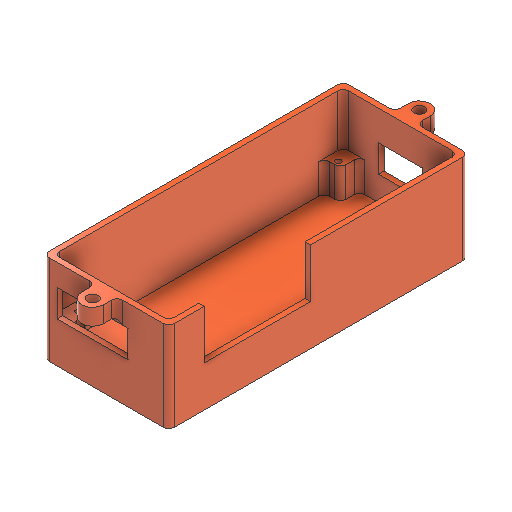
# Autodesk Inventor part: StereoPiBracket
Saved by Autodesk Inventor 2025.2 (Build 292293000, 293)
## iProperties
Created: 2024-08-19
Part Number: StereoPiBracket
Material: Generic
Document SubType Name: Modeling
Designer: 16366081
Density: 1 g/cm^3
Appearance: Default
Author: 16366081
Autodesk Inventor part; units mm, degrees
ref_plane "YZ Plane" through (0, 0, 0) normal (1, 0, 0) x (0, 1, 0)
ref_plane "XZ Plane" through (0, 0, 0) normal (0, 1, 0) x (-1, 0, 0)
ref_plane "XY Plane" through (0, 0, 0) normal (0, 0, 1) x (1, 0, 0)
sketch "Sketch1" plane through (0, 0, 0) normal (0, 1, 0) x (-1, 0, 0)
  line L0 (-23, 55) -> (23, 55)
  line L1 (23, 55) -> (23, -55)
  line L2 (23, -55) -> (-23, -55)
  line L3 (-23, -55) -> (-23, 55)
  line L4 (-23, 55) -> (23, -55) construction
  line L5 (23, 55) -> (-23, -55) construction
  point P0 (0, 0)
  dimension "d0" = 46
  dimension "d1" = 110
  constraints: 12 end point, 2 midpoint, 2 parallel, 1 horizontal, 1 perpendicular
  measures "d0" distance of L1.end L2.end
  measures "d1" distance of L0.end L1.end
extrude "Extrusion1" add sketch "Sketch1" along normal blind 3
sketch "Sketch2" plane through (0, 3, 0) normal (0, 1, 0) x (1, 0, 0)
  line L0 (-23, 55) -> (-23, -55) projected
  line L1 (23, -55) -> (-23, -55)
  line L2 (-23, -55) -> (-23, 55)
  line L3 (-23, 55) -> (23, 55)
  line L4 (23, 55) -> (23, -55)
  line L5 (23, -55) -> (-23, 55) construction
  line L6 (-23, -55) -> (23, 55) construction
  line L7 (21, -53) -> (-21, -53)
  line L8 (-21, -53) -> (-21, 53)
  line L9 (-21, 53) -> (21, 53)
  line L10 (21, 53) -> (21, -53)
  line L11 (21, -53) -> (-21, 53) construction
  line L12 (-21, -53) -> (21, 53) construction
  point P0 (0, 0)
  dimension "d4" = 42
  dimension "d5" = 106
  constraints: 24 end point, 4 midpoint, 4 parallel, 2 horizontal, 2 perpendicular
  measures "d4" distance of L8.end L9.end
  measures "d5" distance of L7.end L8.end
extrude "Extrusion2" add sketch "Sketch2" along normal blind 30
sketch "Sketch5" plane through (0, 33, 0) normal (0, 1, 0) x (1, 0, 0)
  line L0 (23, 55) -> (-23, 55) projected
  line L1 (23, -55) -> (23, 55) projected
  line L2 (-23, 55) -> (-23, -55) projected
  line L3 (21, 53) -> (21, -53) projected
  line L4 (21, -42) -> (23, -42)
  line L5 (23, -42) -> (23, -3)
  line L6 (23, -3) -> (21, -3)
  line L7 (21, -3) -> (21, -42)
  line L8 (-23, -55) -> (23, -55) projected
  point P0 (0, 0)
  point P1 (22, -42)
  point P2 (22, -3)
  dimension "d24" = 13
  dimension "d25" = 58
  constraints: 8 end point, 2 midpoint, 2 parallel, 2 point on line, 1 horizontal, 1 perpendicular
  measures "d24" distance from line of L8 point (22, -42)
  measures "d25" distance from line of L0 point (22, -3)
extrude "Extrusion5" cut sketch "Sketch5" against normal blind 18 contours L1 L4 L3 L6
sketch "Sketch6" plane through (23, 0, -55) normal (0, 0, -1) x (-1, 0, 0)
  line L0 (15, 22) -> (31, 22)
  line L1 (31, 22) -> (31, 12)
  line L2 (31, 12) -> (15, 12)
  line L3 (15, 12) -> (15, 22)
  line L4 (46, 0) -> (46, 33) projected
  line L5 (0, 0) -> (46, 0) projected
  point P0 (23, 0)
  dimension "d28" = 16
  dimension "d29" = 15
  dimension "d30" = 10
  dimension "d32" = 12
  constraints: 8 end point, 2 parallel, 1 horizontal, 1 perpendicular
  measures "d28" distance of L0.start L0.end
  measures "d29" distance from line of L4 L1.end
  measures "d30" distance of L2.end L0.start
  measures "d32" distance between parallel lines of L5 L2
extrude "Extrusion6" cut sketch "Sketch6" against normal blind 15
sketch "Sketch7" plane through (-23, 0, 55) normal (0, 0, 1) x (1, 0, 0)
  line L0 (5, 25) -> (31, 25)
  line L1 (31, 25) -> (31, 15)
  line L2 (31, 15) -> (5, 15)
  line L3 (5, 15) -> (5, 25)
  line L4 (0, 0) -> (0, 33) projected
  line L5 (0, 0) -> (46, 0) projected
  point P0 (23, 0)
  dimension "d35" = 5
  dimension "d36" = 10
  dimension "d37" = 15
  dimension "d38" = 26
  constraints: 8 end point, 2 parallel, 1 horizontal, 1 perpendicular
  measures "d35" distance between parallel lines of L4 L3
  measures "d36" distance of L2.end L0.start
  measures "d37" distance between parallel lines of L5 L2
  measures "d38" distance of L1.end L2.end
extrude "Extrusion7" cut sketch "Sketch7" against normal blind 15
sketch "Sketch9" plane through (0, 33, 0) normal (0, 1, 0) x (1, 0, 0)
  circle A0 centre (0, -60) radius 2
  line L0 (-23, -55) -> (23, -55) projected
  line L1 (4, -55) -> (-4, -55)
  line L2 (-4, -55) -> (-4, -60)
  line L3 (4, -60) -> (4, -55)
  arc A1 (-4, -60) -> (4, -60) centre (0, -60) ccw
  circle A2 centre (0, 60) radius 2
  line L4 (23, 55) -> (-23, 55) projected
  line L5 (4, 55) -> (-4, 55)
  line L6 (-4, 55) -> (-4, 60)
  line L7 (4, 60) -> (4, 55)
  arc A3 (4, 60) -> (-4, 60) centre (0, 60) ccw
  point P0 (0, 0)
  point P1 (0, -55)
  point P2 (0, -55)
  point P3 (0, 55)
  point P4 (0, 55)
  point P5 (0, 55)
  dimension "d77" = 4
  dimension "d78" = 5
  dimension "d79" = 8
  dimension "d80" = 4
  dimension "d81" = 4
  dimension "d82" = 4
  dimension "d83" = 5
  dimension "d84" = 8
  dimension "d85" = 4
  constraints: 12 end point, 5 midpoint, 4 centre point, 4 point on circle, 2 coincident, 2 horizontal, 2 parallel, 2 perpendicular, 2 point on line, 1 tangent, 1 vertical alignment
  measures "d77" diameter of A0
  measures "d78" distance of point (0, -55) A0.centre
  measures "d79" distance of L1.start L1.end
  measures "d80" distance of point (0, -55) L1.start
  measures "d81" radius of A1
  measures "d82" diameter of A2
  measures "d83" distance of point (0, 55) A2.centre
  measures "d84" distance of L5.end L5.start
  measures "d85" distance of L5.start point (0, 55)
extrude "Extrusion10" add sketch "Sketch9" against normal blind 6
fillet "Fillet2" radius 2 6 edges at (-4, 30, -55) (4, 30, -55) (-4, 30, 55) (4, 30, 55) (0, 27, -55) (0, 27, 55)
sketch "Sketch11" plane through (0, 3, 0) normal (0, 1, 0) x (1, 0, 0)
  circle A0 centre (-17.5, 47.75) radius 1
  circle A1 centre (17.5, 47.75) radius 1
  circle A2 centre (-17.5, -47.75) radius 1
  circle A3 centre (17.5, -47.75) radius 1
  line L0 (-21, 53) -> (-21, -53) projected
  line L1 (-21, 53) -> (-15, 53)
  line L2 (-15, 53) -> (-15, 46)
  line L3 (-15, 46) -> (-21, 46)
  line L4 (-21, 46) -> (-21, 53)
  line L5 (21, 53) -> (-21, 53) projected
  line L6 (21, 53) -> (15, 53)
  line L7 (15, 53) -> (15, 46)
  line L8 (15, 46) -> (21, 46)
  line L9 (21, 46) -> (21, 53)
  line L10 (-21, -53) -> (-15, -53)
  line L11 (-15, -53) -> (-15, -46)
  line L12 (-15, -46) -> (-21, -46)
  line L13 (-21, -46) -> (-21, -53)
  line L14 (21, -53) -> (15, -53)
  line L15 (15, -53) -> (15, -46)
  line L16 (15, -46) -> (21, -46)
  line L17 (21, -46) -> (21, -53)
  point P0 (0, 0)
  dimension "d95" = 2
  dimension "d96" = 2
  dimension "d97" = 2
  dimension "d98" = 2
  dimension "d99" = 95.5
  dimension "d100" = 35
  dimension "d101" = 47.75
  dimension "d102" = 17.5
  dimension "d103" = 6
  dimension "d104" = 7
  dimension "d105" = 6
  dimension "d106" = 7
  dimension "d107" = 6
  dimension "d108" = 7
  dimension "d109" = 6
  dimension "d110" = 7
  constraints: 32 end point, 8 parallel, 4 centre point, 4 horizontal, 4 perpendicular, 2 horizontal alignment, 2 point on line, 2 vertical alignment
  measures "d95" diameter of A0
  measures "d96" diameter of A1
  measures "d97" diameter of A2
  measures "d98" diameter of A3
  measures "d99" distance of A3.centre A1.centre
  measures "d100" distance of A1.centre A0.centre
  measures "d101" vertical distance of point (0, 0) A3.centre
  measures "d102" horizontal distance of point (0, 0) A3.centre
  measures "d103" distance of L2.end L3.end
  measures "d104" distance of L1.end L2.end
  measures "d105" distance of L8.end L7.end
  measures "d106" distance of L7.end L6.end
  measures "d107" distance of L12.end L11.end
  measures "d108" distance of L11.end L10.end
  measures "d109" distance of L15.end L16.end
  measures "d110" distance of L14.end L15.end
extrude "Extrusion11" add sketch "Sketch11" along normal blind 11
fillet "Fillet6" radius 2 20 edges at (-23, 16.5, -55) (-23, 16.5, 55) (23, 16.5, 55) (23, 16.5, -55) (21, 23.5, -53) (-21, 23.5, -53) (-21, 23.5, 53) (21, 23.5, 53) (15, 8.5, -46) (-15, 8.5, -46) (15, 8.5, 46) (-15, 8.5, 46) (21, 8.5, -46) (15, 8.5, -53) (-15, 8.5, -53) (-21, 8.5, -46) (-21, 8.5, 46) (-15, 8.5, 53) (21, 8.5, 46) (15, 8.5, 53)
body "Solid1"
